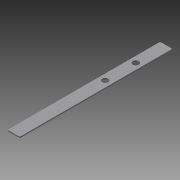
# Autodesk Inventor part: ConnectorStrip
Saved by Autodesk Inventor 2015 (Build 190159000, 159)
## iProperties
Created: 2015-04-17
Part Number: ConnectorStrip
Material: Generic
Document SubType Name: Modeling
Designer: krosie
Density: 1 g/cm^3
Appearance: Default
Author: krosie
Autodesk Inventor part; units mm, degrees
ref_plane "YZ Plane" through (0, 0, 0) normal (1, 0, 0) x (0, 1, 0)
ref_plane "XZ Plane" through (0, 0, 0) normal (0, 1, 0) x (-1, 0, 0)
ref_plane "XY Plane" through (0, 0, 0) normal (0, 0, 1) x (1, 0, 0)
sketch "Sketch1" plane through (0, 0, 0) normal (0, 1, 0) x (-1, 0, 0)
  line L0 (0, 0) -> (10, 0)
  line L1 (10, 0) -> (10, -125)
  line L2 (10, -125) -> (0, -125)
  line L3 (0, -125) -> (0, 0)
  line L4 (27.7651, -45) -> (-20.7182, -45) construction
  circle A0 centre (5, -100) radius 2.5
  circle A1 centre (5, -75) radius 2.5
  point P0 (5, -13.5)
  dimension "d0" = 125
  dimension "d1" = 10
  dimension "d2" = 25
  dimension "d3" = 25
  dimension "d4" = 80
  dimension "d7" = 5
  dimension "d9" = 5
  dimension "d11" = 31.5
  constraints: 10 end point, 2 centre point, 2 coincident, 2 horizontal, 2 parallel, 1 perpendicular
  measures "d0" distance of L0.end L1.end
  measures "d1" distance of L1.end L2.end
  measures "d2" distance from line of L2 point (5, -100)
  measures "d3" distance of point (5, -75) point (5, -100)
  measures "d4" distance between parallel lines of L2 L4
  measures "d7" distance from line of point (5, -75) L1
  measures "d9" diameter of A0
  measures "d11" distance from line of point (5, -13.5) L4
extrude "Extrusion1" add sketch "Sketch1" along normal blind 1
fillet "Fillet1" radius 1 1 edges at (0, 0.5, -125)
fillet "Fillet2" radius 1 3 edges at (0, 0.5, 0) (-10, 0.5, 0) (-10, 0.5, -125)
body "Solid1"
